Autodesk Fusion 360 part; units mm, degrees
note: some values were not read from the file. Chosen so that the rebuilt part matches the saved one: which bodies a step acts on; which face or edge a step refers to; that a step has no effect. Set by a fixed rule: which sketch regions a step uses.
(part 2 of 2)
sketch "Sketch19" plane through (0, -72, 0) normal (0, -1, 0) x (1, 0, 0)
  line L0 (-266, 255) -> (-200.25, 255)
  line L1 (-200.25, 255) -> (-200.25, 178.6667)
  line L2 (-200.25, 178.6667) -> (-263, 178.6667)
  line L3 (-263, 178.6667) -> (-263, 158.2497)
  line L4 (-263, 158.2497) -> (-266, 158.2497)
  line L5 (-266, 158.2497) -> (-266, 129)
  line L6 (-266, 129) -> (-263, 129)
  line L7 (-263, 129) -> (-263, 137.5)
  line L8 (-263, 137.5) -> (-200.25, 137.5)
  line L9 (-200.25, 137.5) -> (-200.25, 61.1667)
  line L10 (-200.25, 61.1667) -> (-263, 61.1667)
  line L11 (-263, 61.1667) -> (-263, 32.25)
  line L12 (-263, 32.25) -> (-266, 32.25)
  line L13 (-266, 32.25) -> (-266, 0)
  line L14 (-266, 0) -> (-260, 0)
  arc A0 (-240, 20) -> (-260, 0) centre (-240, 0) ccw
  line L15 (-240, 20) -> (-26, 20)
  arc A1 (-6, 0) -> (-26, 20) centre (-26, 0) ccw
  line L16 (-6, 0) -> (0, 0)
  line L17 (0, 0) -> (0, 32.25)
  line L18 (0, 32.25) -> (-3, 32.25)
  line L19 (-3, 32.25) -> (-3, 61.1667)
  line L20 (-3, 61.1667) -> (-65.75, 61.1667)
  line L21 (-65.75, 61.1667) -> (-65.75, 137.5)
  line L22 (-65.75, 137.5) -> (-3, 137.5)
  line L23 (-3, 137.5) -> (-3, 129)
  line L24 (-3, 129) -> (0, 129)
  line L25 (0, 129) -> (0, 158.25)
  line L26 (0, 158.25) -> (-3, 158.25)
  line L27 (-3, 158.25) -> (-3, 178.6667)
  line L28 (-3, 178.6667) -> (-65.75, 178.6667)
  line L29 (-65.75, 178.6667) -> (-65.75, 255)
  line L30 (-65.75, 255) -> (-3, 255)
  line L31 (-3, 255) -> (-3, 258)
  line L32 (-3, 258) -> (-266, 258)
  line L33 (-266, 258) -> (-266, 255)
  line L34 (-134.5, 137.5) -> (-134.5, 61.1667)
  line L35 (-134.5, 61.1667) -> (-197.25, 61.1667)
  line L36 (-197.25, 61.1667) -> (-197.25, 137.5)
  line L37 (-197.25, 137.5) -> (-134.5, 137.5)
  line L38 (-68.75, 255) -> (-68.75, 178.6667)
  line L39 (-68.75, 178.6667) -> (-131.5, 178.6667)
  line L40 (-131.5, 178.6667) -> (-131.5, 255)
  line L41 (-131.5, 255) -> (-68.75, 255)
  line L42 (-134.5, 255) -> (-134.5, 178.6667)
  line L43 (-134.5, 178.6667) -> (-197.25, 178.6667)
  line L44 (-197.25, 178.6667) -> (-197.25, 255)
  line L45 (-197.25, 255) -> (-134.5, 255)
  line L46 (-68.75, 137.5) -> (-68.75, 61.1667)
  line L47 (-68.75, 61.1667) -> (-131.5, 61.1667)
  line L48 (-131.5, 61.1667) -> (-131.5, 137.5)
  line L49 (-131.5, 137.5) -> (-68.75, 137.5)
  line L50 (-3, 255) -> (-266, 255)
  dimension "d196" = -3
extrude "Extrude35" cut sketch "Sketch19" against normal blind 10 contours L0 L30 L31 L32 L33 L41 L45 L50 bodies 2
extrude "Extrude36" add 1 faces at (-264, -70, 255) along direction (0, 0, 1) blind 3 on bodies 37 bodies 37
extrude "Extrude37" add 1 faces at (-265, -30.6667, 255) along direction (0, 0, 1) blind 3 separate body on bodies 37 makes body 42
move_body "Move32" bodies 42 to x (1, 0, 0) y (0, 1, 0) z (0, 0, 1) at (65.75, 0, 0)
extrude "Extrude38" cut 1 faces at (-199.25, -30.6667, 258) along direction (0, 0, -1) blind 3 on bodies 42 bodies 6
copy_body "CopyPasteBodies1" bodies 42 makes body 43
move_body "Move33" bodies 43 to x (1, 0, 0) y (0, 1, 0) z (0, 0, 1) at (115, 0, 0)
copy_body "CopyPasteBodies2" bodies 42 makes body 44
move_body "Move34" bodies 44 to x (1, 0, 0) y (0, 1, 0) z (0, 0, 1) at (40, 0, 0)
move_body "Move35" bodies 44 to x (1, 0, 0) y (0, 1, 0) z (0, 0, 1) at (25.75, 0, 0)
move_body "Move36" bodies 43 to x (1, 0, 0) y (0, 1, 0) z (0, 0, 1) at (16.5, 0, 0)
combine "Combine10" operation add target body 8 tool bodies 42
combine "Combine11" operation add target body 7 tool bodies 44
combine "Combine12" operation add target body 9 tool bodies 43
extrude "Extrude39" cut 2 faces at (-133.5, -30.6667, 258) (-67.75, -30.6667, 258) along direction (0, 0, -1) blind 3 on bodies 7 9 bodies 6
extrude "Extrude40" add 1 faces at (0, -30.6667, 257) along direction (1, 0, 0) blind 3 separate body on bodies 6 makes body 45
move_body "Move37" bodies 45 to x (1, 0, 0) y (0, 1, 0) z (0, 0, 1) at (0, 0, -117.5)
move_body "Move38" bodies 45 to x (1, 0, 0) y (0, 1, 0) z (0, 0, 1) at (-3, 0, 0)
extrude "Extrude41" cut 1 faces at (0, -30.6667, 138.5) along direction (-1, 0, 0) blind 3 on bodies 45 bodies 11
copy_body "CopyPasteBodies3" bodies 45 makes body 46
move_body "Move39" bodies 46 to x (1, 0, 0) y (0, 1, 0) z (0, 0, 1) at (-270, 0, 0)
move_body "Move40" bodies 46 to x (1, 0, 0) y (0, 1, 0) z (0, 0, 1) at (7, 0, 0)
extrude "Extrude42" cut 1 faces at (-266, -30.6667, 138.5) along direction (1, 0, 0) blind 3 on bodies 46 bodies 37
ref_plane "WorkPlane11" through (-100.125, -36, 137.5) normal (0, 0, -1) x (1, 0, 0)
split "Split9" by plane through (-100.125, -36, 137.5) normal (0, 0, -1) bodies 10 makes body 47 at (-197.25, -25, 73.8889) makes body 48 at (-131.5, -25, 73.8889) makes body 49 at (-65.75, -25, 73.8889)
mirror "Mirror4" about plane through (-263, -69, 255) normal (0, 0, -1) of bodies 6 makes body 50
move_body "Move41" bodies 50 to x (1, 0, 0) y (0, 1, 0) z (0, 0, 1) at (0, 0, -260)
move_body "Move42" bodies 50 to x (1, 0, 0) y (0, 1, 0) z (0, 0, 1) at (0, 0, 28)
delete_body "RemoveBody10" bodies 1
sketch "Sketch20" plane through (0, 0, 20) normal (0, 0, -1) x (1, 0, 0)
  line L0 (-134.5, 52) -> (-131.5, 52)
  line L1 (-131.5, 52) -> (-131.5, 20)
  line L2 (-131.5, 20) -> (-134.5, 20)
  line L3 (-134.5, 20) -> (-134.5, 52)
  line L4 (-68.75, 52) -> (-65.75, 52)
  line L5 (-65.75, 52) -> (-65.75, 20)
  line L6 (-65.75, 20) -> (-68.75, 20)
  line L7 (-68.75, 20) -> (-68.75, 52)
  line L8 (-200.25, 52) -> (-197.25, 52)
  line L9 (-197.25, 52) -> (-197.25, 20)
  line L10 (-197.25, 20) -> (-200.25, 20)
  line L11 (-200.25, 20) -> (-200.25, 52)
  line L12 (-263, 72) -> (-263, 52)
  line L13 (-263, 52) -> (-266, 52)
  line L14 (-266, 52) -> (-266, 20)
  line L15 (-266, 20) -> (-263, 20)
  line L16 (-263, 20) -> (-263, 3)
  line L17 (-263, 3) -> (-236.45, 3)
  line L18 (-236.45, 3) -> (-236.45, 0)
  line L19 (-236.45, 0) -> (-206.9, 0)
  line L20 (-206.9, 0) -> (-206.9, 3)
  line L21 (-206.9, 3) -> (-177.35, 3)
  line L22 (-177.35, 3) -> (-177.35, 0)
  line L23 (-177.35, 0) -> (-147.8, 0)
  line L24 (-147.8, 0) -> (-147.8, 3)
  line L25 (-147.8, 3) -> (-118.25, 3)
  line L26 (-118.25, 3) -> (-118.25, 0)
  line L27 (-118.25, 0) -> (-88.7, 0)
  line L28 (-88.7, 0) -> (-88.7, 3)
  line L29 (-88.7, 3) -> (-59.15, 3)
  line L30 (-59.15, 3) -> (-59.15, 0)
  line L31 (-59.15, 0) -> (-29.6, 0)
  line L32 (-29.6, 0) -> (-29.6, 3)
  line L33 (-29.6, 3) -> (-3, 3)
  line L34 (-3, 3) -> (-3, 20)
  line L35 (-3, 20) -> (0, 20)
  line L36 (0, 20) -> (0, 52)
  line L37 (0, 52) -> (-3, 52)
  line L38 (-3, 52) -> (-3, 72)
  line L39 (-3, 72) -> (-263, 72)
extrude "Extrude43" add sketch "Sketch20" against normal blind 3 separate body contours L0 L1 L2 L3 | L4 L5 L6 L7 | L8 L9 L10 L11 makes body 51 at (-197.25, -41.3333, 21) makes body 52 at (-131.5, -41.3333, 21) makes body 53 at (-65.75, -41.3333, 21)
combine "Combine13" operation add target body 53 tool bodies 49
combine "Combine14" operation add target body 52 tool bodies 48
combine "Combine15" operation add target body 51 tool bodies 47
extrude "Extrude44" cut 1 faces at (0, -30.6667, 21) along direction (-1, 0, 0) blind 3 on bodies 50 bodies 11
extrude "Extrude45" cut 1 faces at (-266, -30.6667, 22) along direction (1, 0, 0) blind 3 on bodies 50 bodies 37
combine "Combine16" operation add target body 46 tool bodies 10 45
extrude "Extrude46" cut 4 faces at (-39.45, 0, 21) (-108.4, 0, 22) (-226.6, 0, 22) (-167.5, 0, 22) along direction (0, -1, 0) blind 20 on bodies 50 bodies 3
copy_body "CopyPasteBodies4" bodies 6 makes body 54
move_body "Move43" bodies 54 to x (1, 0, 0) y (0, 1, 0) z (0, 0, 1) at (0, 0, -70)
move_body "Move44" bodies 54 to x (1, 0, 0) y (0, 1, 0) z (0, 0, 1) at (0, 0, -47.5)
delete_body "RemoveBody11" bodies 46
extrude "Extrude47" cut 1 faces at (-89.6667, -72, 138.5) along direction (0, 1, 0) blind 3 on bodies 54 bodies 54
extrude "Extrude48" cut 1 faces at (-89.6667, -72, 22) along direction (0, 1, 0) blind 3 on bodies 50 bodies 50
extrude "Extrude49" cut 4 faces at (-39.45, 0, 139.5) (-108.4, 0, 138.5) (-167.5, 0, 138.5) (-226.6, 0, 138.5) along direction (0, -1, 0) blind 3 on bodies 54 bodies 3
sketch "Sketch21" plane through (0, 0, 140.5) normal (0, 0, 1) x (-1, 0, 0)
  line L0 (263, 69) -> (3, 69)
  line L1 (3, 69) -> (3, 52)
  line L2 (3, 52) -> (0, 52)
  line L3 (0, 52) -> (0, 20)
  line L4 (0, 20) -> (3, 20)
  line L5 (3, 20) -> (3, 3)
  line L6 (3, 3) -> (29.6, 3)
  line L7 (29.6, 3) -> (29.6, 0)
  line L8 (29.6, 0) -> (59.15, 0)
  line L9 (59.15, 0) -> (59.15, 3)
  line L10 (59.15, 3) -> (88.7, 3)
  line L11 (88.7, 3) -> (88.7, 0)
  line L12 (88.7, 0) -> (118.25, 0)
  line L13 (118.25, 0) -> (118.25, 3)
  line L14 (118.25, 3) -> (147.8, 3)
  line L15 (147.8, 3) -> (147.8, 0)
  line L16 (147.8, 0) -> (177.35, 0)
  line L17 (177.35, 0) -> (177.35, 3)
  line L18 (177.35, 3) -> (206.9, 3)
  line L19 (206.9, 3) -> (206.9, 0)
  line L20 (206.9, 0) -> (236.45, 0)
  line L21 (236.45, 0) -> (236.45, 3)
  line L22 (236.45, 3) -> (263, 3)
  line L23 (263, 3) -> (263, 20)
  line L24 (263, 20) -> (266, 20)
  line L25 (266, 20) -> (266, 52)
  line L26 (266, 52) -> (263, 52)
  line L27 (263, 52) -> (263, 69)
  line L28 (197.25, 52) -> (200.25, 52)
  line L29 (200.25, 52) -> (200.25, 20)
  line L30 (200.25, 20) -> (197.25, 20)
  line L31 (197.25, 20) -> (197.25, 52)
  line L32 (65.75, 52) -> (68.75, 52)
  line L33 (68.75, 52) -> (68.75, 20)
  line L34 (68.75, 20) -> (65.75, 20)
  line L35 (65.75, 20) -> (65.75, 52)
  line L36 (131.5, 52) -> (134.5, 52)
  line L37 (134.5, 52) -> (134.5, 20)
  line L38 (134.5, 20) -> (131.5, 20)
  line L39 (131.5, 20) -> (131.5, 52)
extrude "Extrude50" add sketch "Sketch21" against normal blind 1.5 separate body contours L28 L29 L30 L31 | L32 L33 L34 L35 | L36 L37 L38 L39 makes body 55 at (-199.25, -30.6667, 140.5) makes body 56 at (-133.5, -30.6667, 140.5) makes body 57 at (-67.75, -30.6667, 140.5)
combine "Combine17" operation add target body 55 tool bodies 8
combine "Combine18" operation add target body 56 tool bodies 7
combine "Combine19" operation add target body 57 tool bodies 9
sketch "Sketch22" plane through (0, 0, 137.5) normal (0, 0, -1) x (1, 0, 0)
  line L0 (-3, 69) -> (-263, 69)
  line L1 (-263, 69) -> (-263, 52)
  line L2 (-263, 52) -> (-266, 52)
  line L3 (-266, 52) -> (-266, 20)
  line L4 (-266, 20) -> (-263, 20)
  line L5 (-263, 20) -> (-263, 3)
  line L6 (-263, 3) -> (-236.45, 3)
  line L7 (-236.45, 3) -> (-236.45, 0)
  line L8 (-236.45, 0) -> (-206.9, 0)
  line L9 (-206.9, 0) -> (-206.9, 3)
  line L10 (-206.9, 3) -> (-177.35, 3)
  line L11 (-177.35, 3) -> (-177.35, 0)
  line L12 (-177.35, 0) -> (-147.8, 0)
  line L13 (-147.8, 0) -> (-147.8, 3)
  line L14 (-147.8, 3) -> (-118.25, 3)
  line L15 (-118.25, 3) -> (-118.25, 0)
  line L16 (-118.25, 0) -> (-88.7, 0)
  line L17 (-88.7, 0) -> (-88.7, 3)
  line L18 (-88.7, 3) -> (-59.15, 3)
  line L19 (-59.15, 3) -> (-59.15, 0)
  line L20 (-59.15, 0) -> (-29.6, 0)
  line L21 (-29.6, 0) -> (-29.6, 3)
  line L22 (-29.6, 3) -> (-3, 3)
  line L23 (-3, 3) -> (-3, 20)
  line L24 (-3, 20) -> (0, 20)
  line L25 (0, 20) -> (0, 52)
  line L26 (0, 52) -> (-3, 52)
  line L27 (-3, 52) -> (-3, 69)
  line L28 (-134.5, 52) -> (-131.5, 52)
  line L29 (-131.5, 52) -> (-131.5, 20)
  line L30 (-131.5, 20) -> (-134.5, 20)
  line L31 (-134.5, 20) -> (-134.5, 52)
  line L32 (-68.75, 52) -> (-65.75, 52)
  line L33 (-65.75, 52) -> (-65.75, 20)
  line L34 (-65.75, 20) -> (-68.75, 20)
  line L35 (-68.75, 20) -> (-68.75, 52)
  line L36 (-200.25, 52) -> (-197.25, 52)
  line L37 (-197.25, 52) -> (-197.25, 20)
  line L38 (-197.25, 20) -> (-200.25, 20)
  line L39 (-200.25, 20) -> (-200.25, 52)
extrude "Extrude51" add sketch "Sketch22" against normal blind 1.5 separate body contours L28 L29 L30 L31 | L32 L33 L34 L35 | L36 L37 L38 L39 makes body 58 at (-66.75, -30.6667, 137.5) makes body 59 at (-132.5, -30.6667, 137.5) makes body 60 at (-198.25, -30.6667, 137.5)
combine "Combine20" operation add target body 60 tool bodies 51
combine "Combine21" operation add target body 52 tool bodies 59
combine "Combine22" operation add target body 53 tool bodies 58
equation "d1 = width"
equation "polycarbonateThickness = 3 mm" comment "Thickness of the polycarbonate panels"
equation "d3 = polycarbonateThickness"
equation "collectorWidth = ( width - 5 * polycarbonateThickness ) / 4" comment "Width of a Smartie collector"
equation "d37 = collectorLength - polycarbonateThickness"
equation "collectorHeight = ( height - 3 * polycarbonateThickness - bottomHeight ) / 2" comment "Height of a Smartie Collector"
equation "height = 262 mm - tolerance" comment "Height of the Sorted Smarties Collector"
equation "d41 = height"
equation "bottomHeight = 20 mm" comment "Heigh of the botom part of the Sorted Smarties Collector"
equation "d51 = polycarbonateThickness"
equation "d52 = polycarbonateThickness"
equation "d53 = polycarbonateThickness"
equation "d54 = bottomHeight"
equation "d55 = polycarbonateThickness"
equation "d56 = polycarbonateThickness"
equation "d57 = polycarbonateThickness"
equation "d58 = polycarbonateThickness"
equation "d59 = polycarbonateThickness"
equation "d60 = collectorHeight"
equation "d62 = collectorWidth"
equation "d63 = collectorWidth"
equation "d64 = collectorWidth"
equation "d66 = polycarbonateThickness"
equation "d67 = -width"
equation "d69 = -polycarbonateThickness"
equation "openingHeight = collectorHeight * 2 / 3" comment "Height of the open part at the front of the Smartie collectors"
equation "d72 = openingHeight"
equation "d73 = openingHeight"
equation "d74 = -collectorLength"
equation "collectorLength = 72 mm" comment "Depth of the Sorted Smarties Collector Component"
equation "d80 = 2 * polycarbonateThickness + 20 mm"
equation "d81 = 2 * polycarbonateThickness + 20 mm"
equation "tolerance = 4 mm" comment "Tolerance to allow for easy motion"
equation "width = 270 mm - tolerance" comment "Width of the Sorted Smarties Component"
equation "d84 = collectorWidth"
equation "d85 = collectorWidth"
equation "d86 = collectorWidth"
equation "d87 = collectorWidth"
equation "d88 = collectorWidth"
equation "d89 = collectorWidth"
equation "d90 = collectorWidth"
equation "d91 = collectorWidth"
named bodies: "Sorted Smarties Collector", "Sorted Smarties Collector (1)", "Sorted Smarties Collector (2)", "Sorted Smarties Collector (3)", "Sorted Smarties Collector (4)", "Sorted Smarties Collector (5)", "Sorted Smarties Collector (6)", "Sorted Smarties Collector (7)", "Sorted Smarties Collector (8)", "Sorted Smarties Collector (9)", "Sorted Smarties Collector (1) (1)", "Sorted Smarties Collector (1) (2)", "Sorted Smarties Collector (1) (1) (1)", "Sorted Smarties Collector (1) (1) (1) (1)", "Sorted Smarties Collector (1) (1) (2)", "Sorted Smarties Collector (9) (1)", "Sorted Smarties Collector (9) (2)", "Sorted Smarties Collector (9) (3)", "Sorted Smarties Collector (5) (1)", "Sorted Smarties Collector (5) (2)"
